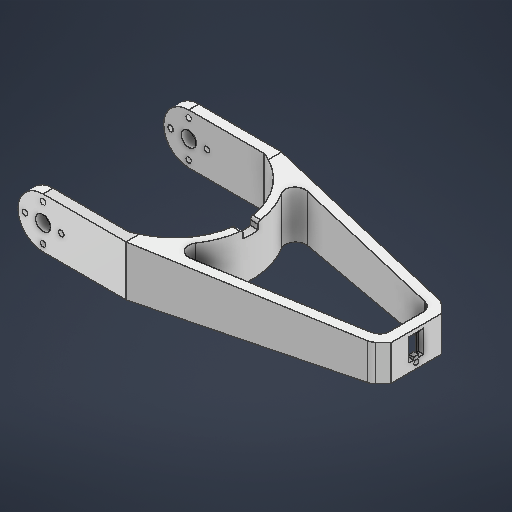
# Autodesk Inventor part: calf_2
Saved by Autodesk Inventor 2026.1 (Build 301233000, 233)
## iProperties
Created: 2025-08-26
Part Number: calf_2
Material: Generic
Document SubType Name: Modeling
Designer: emanuel
Density: 1 g/cm^3
Appearance: Default
Author: emanuel
Autodesk Inventor part; units mm, degrees
ref_plane "YZ Plane" through (0, 0, 0) normal (1, 0, 0) x (0, 1, 0)
ref_plane "XZ Plane" through (0, 0, 0) normal (0, 1, 0) x (-1, 0, 0)
ref_plane "XY Plane" through (0, 0, 0) normal (0, 0, 1) x (1, 0, 0)
sketch "Sketch1" plane through (0, 0, 0) normal (0, 1, 0) x (-1, 0, 0)
  line L0 (0, 0) -> (0, -54)
  line L1 (0, -54) -> (5, -54)
  line L2 (5, -54) -> (5, -58)
  line L3 (5, -58) -> (0, -58)
  line L4 (0, -58) -> (0, -54)
  line L5 (0, 0) -> (3, 0)
  line L6 (3, 0) -> (3, 4)
  line L7 (3, 4) -> (0, 4)
  line L8 (0, 4) -> (0, 0)
  line L9 (3, 0) -> (0, 0)
  line L10 (0, 0) -> (0, -54)
  line L11 (0, -54) -> (3, -54)
  line L12 (3, -54) -> (3, 0)
  line L13 (3, 4) -> (43, 4)
  line L14 (43, 4) -> (43, 0)
  line L15 (43, 0) -> (3, 0)
  line L16 (3, 0) -> (3, 4)
  line L17 (3, -54) -> (43, -54)
  line L18 (43, -54) -> (43, -58)
  line L19 (43, -58) -> (3, -58)
  line L20 (3, -58) -> (3, -54)
  line L21 (0, -27) -> (-82.8143, -27)
  line L22 (-82.8143, -27) -> (-97.578, -27)
  line L23 (0, 4) -> (90, 4) construction
  line L24 (0, 0) -> (80, 0) construction
  line L25 (-84.5723, -27) -> (-84.5723, -17)
  line L26 (-84.5723, -27) -> (-84.5723, -37)
  line L27 (-84.5723, -37) -> (-80.5723, -37)
  line L28 (-80.5723, -37) -> (-80.5723, -17)
  line L29 (-80.5723, -17) -> (-84.5723, -17)
  line L30 (0, 0) -> (-80.5723, -17)
  line L31 (0, -54) -> (-80.5723, -37)
  line L32 (-80.5723, -37) -> (-80.5723, -41)
  line L33 (-80.5723, -41) -> (0, -58)
  line L34 (-84.5723, -37) -> (-80.5723, -41)
  line L35 (-80.5723, -17) -> (-80.5723, -13)
  line L36 (-80.5723, -13) -> (0, 4)
  line L37 (-84.5723, -17) -> (-80.5723, -13)
  line L38 (3, -27) -> (13, -27)
  circle A0 centre (13, -27) radius 28.7924
  line L39 (41.7924, -27) -> (44.7924, -27)
  circle A1 centre (13, -27) radius 31.7924
  point P0 (-85.1718, -27)
  point P1 (-74.1819, -27)
  point P2 (3, 0)
  point P3 (-5.5314, -1.1671)
  point P4 (-5.5314, -52.8329)
  dimension "d0" = 54
  dimension "d1" = 5
  dimension "d2" = 4
  dimension "d3" = 3
  dimension "d4" = 4
  dimension "d5" = 40
  dimension "d6" = 40
  dimension "d32" = 10
  dimension "d34" = 10
  dimension "d35" = 4
  dimension "d36" = 4
  dimension "d37" = 4
  dimension "d41" = 10
  dimension "d42" = 3
  dimension "d58" = 4
  constraints: 80 end point, 10 horizontal, 10 parallel, 9 point on line, 8 perpendicular, 3 vertical, 2 coincident, 2 midpoint, 2 point on circle, 1 centre point, 3 other
  measures "d0" distance of L0.start L0.end
  measures "d1" distance of L2.end L3.end
  measures "d2" distance of L1.end L2.end
  measures "d3" distance of L7.end L6.end
  measures "d4" distance of L6.end L5.end
  measures "d5" distance of L14.end L15.end
  measures "d6" distance of L18.end L19.end
  measures "d32" distance of L25.start L25.end
  measures "d34" distance of L25.start L26.end
  measures "d35" distance of L26.end L27.end
  measures "d36" distance of L27.end L32.end
  measures "d37" distance of L28.end L35.end
  measures "d41" distance of L38.start L38.end
  measures "d42" distance of L39.start L39.end
  measures "d58" distance between parallel lines of L25 L28
extrude "Extrusion1" add sketch "Sketch1" along normal blind 20 contours L5 A0 L0 | L8 A1 L6 L5 | L30 A1 L8 | L0 A0 L21 A1 L30 | A0 L15 | L6 A1 L13 L15 A0 | A1 L30 L35 L36 L8 | L8 L7 L6 A1 | A0 L0 L31 A1 L21 | L6 L13 A1 | L28 L21 L22 L25 L29 | L29 L37 L35 | A0 L1 L0 | L20 A1 L4 L1 | A0 L2 A1 L20 | L1 L2 A0 | A1 L13 L14 L15 | L28 L27 L26 L22 L21 | A1 L4 L33 L32 L31 | L31 L4 A1 | L17 A0 L2 | A1 L2 L3 L20 | L20 L3 L4 A1 | A0 L17 A1 L19 L2 | L32 L34 L27 | A1 L19 L2 | L17 L18 L19 A1
sketch "Sketch2" plane through (-43, 0, 4) normal (0, 0, 1) x (1, 0, 0)
  line L0 (43, 20) -> (0, 20) projected
  line L1 (0, 20) -> (10, 20)
  line L2 (10, 20) -> (10, 10)
  line L3 (10, 10) -> (0, 10)
  line L4 (0, 10) -> (0, 20)
  circle A0 centre (10, 10) radius 3
  circle A1 centre (10, 10) radius 10
  line L5 (128.1718, 0) -> (128.1718, 20) projected
  line L6 (128.1718, 10) -> (128.1718, 17)
  line L7 (128.1718, 17) -> (128.1718, 3)
  line L8 (43, 0) -> (0, 0) projected
  line L9 (128.1718, 3) -> (43, 0)
  line L10 (43, 0) -> (128.1718, 0)
  line L11 (128.1718, 0) -> (128.1718, 3)
  line L12 (43, 20) -> (73.6773, 20) projected
  line L13 (128.1718, 17) -> (43, 20)
  line L14 (128.1718, 20) -> (43, 20) projected
  line L15 (43, 20) -> (128.1718, 20)
  line L16 (128.1718, 20) -> (128.1718, 17)
  line L17 (10, 10) -> (0, 10)
  line L18 (0, 10) -> (0, 0)
  line L19 (0, 0) -> (10, 0)
  line L20 (10, 0) -> (10, 10)
  circle A2 centre (10, 10) radius 8
  circle A3 centre (10, 10) radius 6.5
  line L21 (10, 18) -> (10, 16.5)
  circle A4 centre (10, 17.25) radius 1.1
  line L22 (2, 10) -> (3.5, 10)
  circle A5 centre (2.75, 10) radius 1.1
  line L23 (10, 3.5) -> (10, 2)
  circle A6 centre (10, 2.75) radius 1.1
  line L24 (16.5, 10) -> (18, 10)
  circle A7 centre (17.25, 10) radius 1.1
  dimension "d15" = 10
  dimension "d16" = 10
  dimension "d17" = 6
  dimension "d18" = 7
  dimension "d19" = 14
  dimension "d22" = 16
  dimension "d23" = 13
  dimension "d24" = 2.2
  dimension "d25" = 2.2
  dimension "d26" = 2.2
  dimension "d27" = 2.2
  constraints: 40 end point, 8 point on circle, 8 point on line, 7 centre point, 5 midpoint, 5 parallel, 4 coincident, 4 perpendicular, 3 horizontal, 1 collinear, 1 vertical, 3 other
  measures "d15" distance of L2.end L3.end
  measures "d16" distance of L1.end L2.end
  measures "d17" diameter of A0
  measures "d18" distance of L6.start L6.end
  measures "d19" distance of L6.end L7.end
  measures "d22" diameter of A2
  measures "d23" diameter of A3
  measures "d24" diameter of A4
  measures "d25" diameter of A5
  measures "d26" diameter of A6
  measures "d27" diameter of A7
extrude "Extrusion2" cut sketch "Sketch2" against normal blind 100 contours L12 L14 L5 L13 | A1 L4 L0 | A4 A2 L2 | L2 A2 A4 | A1 L8 L18 | A2 A4 A3 L2 | L2 A3 A4 A2 | A5 A2 L3 | L3 A2 A5 | L5 L10 L9 | A3 A4 L2 | L2 A4 A3 | A7 A2 | A2 L24 A3 A7 | A5 A3 L3 A2 | A6 A2 L20 | L20 A2 A6 | L3 A3 A5 A2 | A2 A7 A3 L24 | A3 A7 | A5 L3 A3 | A2 A6 A3 L20 | L20 A3 A6 A2 | L3 A5 A3 | A0 L20 L2 | L2 L3 A0 | A3 A6 L20 | L20 A6 A3 | L20 A0 L3
sketch "Sketch3" plane through (80.5723, 2.838, -17) normal (-1, 0, 0) x (0, 0, 1)
  line L0 (0, 14.324) -> (-20, 14.324) projected
  line L1 (-20, 14.1831) -> (0, 14.1831) projected
  line L2 (0, 14.324) -> (-20, 14.1831)
  line L3 (-10, 14.2536) -> (-10, 0)
  line L4 (-20, 0) -> (0, 0) projected
  line L5 (-14, 0.6268) -> (-6, 0.6268)
  line L6 (-6, 0.6268) -> (-6, 13.6268)
  line L7 (-6, 13.6268) -> (-14, 13.6268)
  line L8 (-14, 13.6268) -> (-14, 0.6268)
  line L9 (-14, 0.6268) -> (-6, 13.6268) construction
  line L10 (-6, 0.6268) -> (-14, 13.6268) construction
  line L11 (-14, 0.6268) -> (-10, 0.6268)
  line L12 (-10, 0.6268) -> (-10, 2.4268)
  line L13 (-10, 2.4268) -> (-14, 2.4268)
  line L14 (-14, 2.4268) -> (-14, 0.6268)
  circle A0 centre (-10, 2.4268) radius 1
  line L15 (-14, 13.6268) -> (-6, 13.6268)
  line L16 (-6, 13.6268) -> (-6, 12.6268)
  line L17 (-6, 12.6268) -> (-14, 12.6268)
  line L18 (-14, 12.6268) -> (-14, 13.6268)
  line L19 (-14, 13.6268) -> (-13, 13.6268)
  line L20 (-13, 13.6268) -> (-13, 0.6268)
  line L21 (-13, 0.6268) -> (-14, 0.6268)
  line L22 (-14, 0.6268) -> (-14, 13.6268)
  line L23 (-6, 13.6268) -> (-7, 13.6268)
  line L24 (-7, 13.6268) -> (-7, 0.6268)
  line L25 (-7, 0.6268) -> (-6, 0.6268)
  line L26 (-6, 0.6268) -> (-6, 13.6268)
  line L27 (-6, 0.6268) -> (-14, 0.6268)
  line L28 (-14, 0.6268) -> (-14, 3.6268)
  line L29 (-14, 3.6268) -> (-6, 3.6268)
  line L30 (-6, 3.6268) -> (-6, 0.6268)
  line L31 (-9.0365, 2.6944) -> (-11, 2.6944)
  line L32 (-11, 2.6944) -> (-11, 4.6268)
  line L33 (-11, 4.6268) -> (-9.0365, 4.6268)
  line L34 (-9.0365, 4.6268) -> (-9.0365, 2.6944)
  line L35 (-6, 13.6268) -> (-7, 13.6268)
  line L36 (-7, 13.6268) -> (-7, 3.6268)
  line L37 (-7, 3.6268) -> (-6, 3.6268)
  line L38 (-6, 3.6268) -> (-6, 13.6268)
  point P0 (17, -2.838)
  point P1 (-10, 7.1268)
  point P2 (-9.0365, 3.6268)
  point P3 (-7, 12.6268)
  point P4 (-13, 12.6268)
  point P5 (-13, 3.6268)
  point P6 (-11, 3.6268)
  dimension "d46" = 2
  dimension "d38" = 8
  dimension "d39" = 13
  dimension "d44" = 4
  dimension "d45" = 1.8
  dimension "d47" = 1
  dimension "d48" = 1
  dimension "d49" = 1
  dimension "d50" = 3
  dimension "d51" = 4
  constraints: 72 end point, 16 parallel, 8 horizontal, 8 perpendicular, 6 point on line, 5 midpoint, 1 coincident, 3 other
  measures "d38" distance of L7.end L6.end
  measures "d39" distance of L6.end L5.end
  measures "d44" distance of L13.end L12.end
  measures "d45" distance of L12.end L11.end
  measures "d47" distance of L15.end L16.end
  measures "d48" distance of L20.end L21.end
  measures "d49" distance of L25.end L24.end
  measures "d50" distance of L27.end L28.end
  measures "d51" distance between parallel lines of L5 L33
fillet "Fillet1" radius 4 4 edges at (80.5723, 10, -41) (80.5723, 10, -13) (80.5723, 10, -37) (80.5723, 10, -17)
fillet "Fillet2" radius 4 2 edges at (5.5314, 10, -52.8329) (5.5314, 10, -1.1671)
extrude "Extrusion3" cut sketch "Sketch3" against normal blind 20 contours L17 L24 L29 L34 L33 L3 | L3 L33 L32 L29 L20 L17 | A0 L31 L3 | L3 L31 A0 | L31 A0 L3 | L3 L13 A0 L31 | L13 L3 A0
extrude "Extrusion4" cut sketch "Sketch3" against normal blind 2 contours L7 L24 L17 L3 | L3 L17 L20 L7 | L7 L6 L17 L24 | L20 L17 L8 L7 | L33 L34 L29 L3 | L3 L29 L32 L33 | L17 L6 L29 L24 | L20 L29 L8 L17 | L29 L34 A0 L3 | L3 A0 L31 L32 L29 | L29 L6 L5 L24 | L24 L5 L3 A0 L34 L29 | L29 L32 L31 A0 L13 L20 | L20 L13 L8 L29 | A0 L31 L3 | L3 L31 A0 | L20 L5 L8 L13 | L13 A0 L3 L5 L20 | L31 A0 L3 | L3 L13 A0 L31 | L13 L3 A0
sketch "Sketch4" plane through (84.5723, 17.0211, -17) normal (0.0352, 0.9994, 0) x (0.9994, -0.0352, 0)
  ellipse E0 centre (-97.6328, 10) end of major axis (-129.4449, 10) minor radius 31.7924 (-70.8385, -7.1379) -> (-70.8385, 27.1379) ccw projected
  line L0 (-97.6328, 10) -> (-62.4593, 10)
  line L1 (-62.4593, 10) -> (-62.4593, 13)
  line L2 (-62.4593, 13) -> (-97.6328, 13)
  line L3 (-97.6328, 13) -> (-97.6328, 10)
  line L4 (-97.6328, 10) -> (-62.4593, 10)
  line L5 (-62.4593, 10) -> (-62.4593, 7)
  line L6 (-62.4593, 7) -> (-97.6328, 7)
  line L7 (-97.6328, 7) -> (-97.6328, 10)
  point P0 (-83.9208, -17)
  point P1 (-62.4593, 10)
  dimension "d59" = 3
  dimension "d60" = 3
  constraints: 16 end point, 4 parallel, 2 horizontal, 2 perpendicular, 1 point on line, 1 other
  measures "d59" distance of L1.end L0.end
  measures "d60" distance of L4.end L5.end
extrude "Extrusion6" cut sketch "Sketch4" against normal blind 3
fillet "Fillet3" radius 1 2 edges at (17.1431, 19.3962, -30) (17.1431, 19.3962, -24)
body "Solid1"
